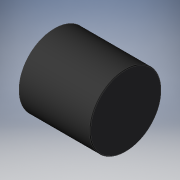
# Autodesk Inventor part: HXNN8-8
Saved by Autodesk Inventor 2019 (Build 230136000, 136)
## iProperties
Created: 2023-11-07
Part Number: HXNN8-8
Material: Generic
Catalog Web Link: www.cadenas.de
Description: HXN, HXNH, HXMS, HXNN-Magnets - Square Round Type
Vendor: MISUMI
Document SubType Name: Modeling
Designer: psAdmin
Manufacturer: MISUMI
Mass: 0.401964 g
Surface Area: 2.99221 cm^2
Volume: 0.401964 cm^3
Density: 1 g/cm^3
Appearance: PSOLRGB-175-175-175
Category: PARTsolutions
Company: MISUMI
Title: HXNN8-8
Author: Cadenas PARTsolutions
Comments: Magnets - Square Round Type
PSOL_IDENT_0: {$CADENAS_DATA/23d-libs/misumi/metric/28_keys_magnets/hxms.prj},175 {VTYP=3D},{NB=HXNN8-8},{LINA=HXN
PSOL_IDENT_1: N8-8},{NN=HXN, HXNH, HXMS, HXNN},{DATE=29.05.2023 07:55:40},{GEOMDATE=16.08.2019 01:12:06},{VERSION=
PSOL_IDENT_2: },{LINEID=50},{WBVAR=MAT,L},{WBNUMERIC=L}  {NB=HXNN8-8},{LINA=HXNN8-8},{KT=DUMMY},{PN=HXNN8-8},{TYPE=
PSOL_IDENT_3: HXNN},{MAT=NN},{MATALG= 'NN', 'Powerful Neodymium Magnet','N', 'Neodymium Magnet', 'NH', 'Heat Resis
PSOL_IDENT_4: tant Neodymium Magnet'  , 'MS', 'Cobalt Magnet' },{ST=Nickel Plating},{HR=60},{D=8},{L=8},{LHXNN=2,3
PSOL_IDENT_5: ,5,6,8,10},{LHXN=2,3,5,6,8,10},{LHXNH=2,3,5,8},{LHXMS=2,3,5,8},{LALG=2,3,5,6,8,10},{COLR=0.00},{COLG=
PSOL_IDENT_6: 0.00},{COLB=1.00},{C=0.08}
NB: HXNN8-8
NN: HXN, HXNH, HXMS, HXNN
NT: Magnets - Square Round Type
NBSYN: $PN.
LINA: HXNN8-8
CATALOG: Misumi
PN: HXNN8-8
MAT: Powerful Neodymium Magnet
ST: Nickel Plating
HR: 60
D: 8
L: 8
SUPPLIER: MISUMI
ARTICLENO: HXNN8-8
BOMINFO: HXNN8-8
CREATOR: CADENAS GmbH
Autodesk Inventor part; units mm, degrees
ref_plane "YZ Plane" through (0, 0, 0) normal (1, 0, 0) x (0, 1, 0)
ref_plane "XZ Plane" through (0, 0, 0) normal (0, 1, 0) x (-1, 0, 0)
ref_plane "XY Plane" through (0, 0, 0) normal (0, 0, 1) x (1, 0, 0)
sketch "Sketch_1" plane through (0, 0, 0) normal (0, 0, 1) x (1, 0, 0)
  line L0 (8, 0) -> (0, 0)
  line L1 (0, 0) -> (0, 3.92)
  line L2 (0, 3.92) -> (0.08, 4)
  line L3 (0.08, 4) -> (7.92, 4)
  line L4 (7.92, 4) -> (8, 3.92)
  line L5 (8, 3.92) -> (8, 0)
  line L6 (8, 0) -> (0, 0)
  constraints: 14 end point
revolve "Revolution1" add sketch "Sketch_1" angle 360 about axis through (8, 0, 0) along (1, 0, 0)
body "Solid1"
